Autodesk Fusion 360 part; units mm, degrees
(part 2 of 2)
sketch "スケッチ3" plane through (0, 0, 1.5) normal (0, 0, 1) x (-1, 0, 0)
  line L0 (-5.6421, -16.3724) -> (-10.7928, -25.2936)
  arc A0 (-10.7928, -25.2936) -> (-3.3, -27.3013) centre (0, 0) ccw
  line L1 (-3.3, -27.3013) -> (-3.3, -17)
  line L2 (-3.3, -17) -> (3.3, -17)
  line L3 (3.3, -17) -> (3.3, -27.3013)
  arc A1 (3.3, -27.3013) -> (10.7928, -25.2936) centre (0, 0) ccw
  line L4 (10.7928, -25.2936) -> (5.6421, -16.3724)
  line L5 (5.6421, -16.3724) -> (11.3579, -13.0724)
  line L6 (11.3579, -13.0724) -> (16.5085, -21.9936)
  arc A2 (16.5085, -21.9936) -> (21.9936, -16.5085) centre (0, 0) ccw
  line L7 (21.9936, -16.5085) -> (13.0724, -11.3579)
  line L8 (13.0724, -11.3579) -> (16.3724, -5.6421)
  line L9 (16.3724, -5.6421) -> (25.2936, -10.7928)
  arc A3 (25.2936, -10.7928) -> (27.3013, -3.3) centre (0, 0) ccw
  line L10 (27.3013, -3.3) -> (17, -3.3)
  line L11 (17, -3.3) -> (17, 3.3)
  line L12 (17, 3.3) -> (27.3013, 3.3)
  arc A4 (27.3013, 3.3) -> (25.2936, 10.7928) centre (0, 0) ccw
  line L13 (25.2936, 10.7928) -> (16.3724, 5.6421)
  line L14 (16.3724, 5.6421) -> (13.0724, 11.3579)
  line L15 (13.0724, 11.3579) -> (21.9936, 16.5085)
  arc A5 (21.9936, 16.5085) -> (16.5085, 21.9936) centre (0, 0) ccw
  line L16 (16.5085, 21.9936) -> (11.3579, 13.0724)
  line L17 (11.3579, 13.0724) -> (5.6421, 16.3724)
  line L18 (5.6421, 16.3724) -> (10.7928, 25.2936)
  arc A6 (10.7928, 25.2936) -> (3.3, 27.3013) centre (0, 0) ccw
  line L19 (3.3, 27.3013) -> (3.3, 17)
  line L20 (3.3, 17) -> (-3.3, 17)
  line L21 (-3.3, 17) -> (-3.3, 27.3013)
  arc A7 (-3.3, 27.3013) -> (-10.7928, 25.2936) centre (0, 0) ccw
  line L22 (-10.7928, 25.2936) -> (-5.6421, 16.3724)
  line L23 (-5.6421, 16.3724) -> (-11.3579, 13.0724)
  line L24 (-11.3579, 13.0724) -> (-16.5085, 21.9936)
  arc A8 (-16.5085, 21.9936) -> (-21.9936, 16.5085) centre (0, 0) ccw
  line L25 (-21.9936, 16.5085) -> (-13.0724, 11.3579)
  line L26 (-13.0724, 11.3579) -> (-16.3724, 5.6421)
  line L27 (-16.3724, 5.6421) -> (-25.2936, 10.7928)
  arc A9 (-25.2936, 10.7928) -> (-27.3013, 3.3) centre (0, 0) ccw
  line L28 (-27.3013, 3.3) -> (-17, 3.3)
  line L29 (-17, 3.3) -> (-17, -3.3)
  line L30 (-17, -3.3) -> (-27.3013, -3.3)
  arc A10 (-27.3013, -3.3) -> (-25.2936, -10.7928) centre (0, 0) ccw
  line L31 (-25.2936, -10.7928) -> (-16.3724, -5.6421)
  line L32 (-16.3724, -5.6421) -> (-13.0724, -11.3579)
  line L33 (-13.0724, -11.3579) -> (-21.9936, -16.5085)
  arc A11 (-21.9936, -16.5085) -> (-16.5085, -21.9936) centre (0, 0) ccw
  line L34 (-16.5085, -21.9936) -> (-11.3579, -13.0724)
  line L35 (-11.3579, -13.0724) -> (-5.6421, -16.3724)
  line L36 (3.3, -27.3013) -> (3.3, -26.1013)
  line L37 (3.3, -26.1013) -> (3.3, -23.5013)
  line L38 (3.3, -23.5013) -> (5.3, -23.5013)
  line L39 (5.3, -23.5013) -> (5.3, -26.1013)
  line L40 (5.3, -26.1013) -> (3.3, -26.1013)
  line L41 (3.3, -26.1013) -> (3.3, -23.5013)
  line L42 (-3.3, -27.3013) -> (-3.3, -26.1013)
  line L43 (-3.3, -26.1013) -> (-5.3, -26.1013)
  line L44 (-5.3, -26.1013) -> (-5.3, -23.5013)
  line L45 (-5.3, -23.5013) -> (-3.3, -23.5013)
  line L46 (-3.3, -23.5013) -> (-3.3, -26.1013)
  line L47 (14.6085, -18.7027) -> (16.3406, -17.7027)
  line L48 (16.3406, -17.7027) -> (17.6406, -19.9544)
  line L49 (17.6406, -19.9544) -> (15.9085, -20.9544)
  line L50 (15.9085, -20.9544) -> (14.6085, -18.7027)
  line L51 (8.8928, -22.0027) -> (10.1928, -24.2544)
  line L52 (7.1607, -23.0027) -> (8.8928, -22.0027)
  line L53 (8.4607, -25.2544) -> (7.1607, -23.0027)
  line L54 (10.1928, -24.2544) -> (8.4607, -25.2544)
  line L55 (22.0027, -8.8928) -> (23.0027, -7.1607)
  line L56 (23.0027, -7.1607) -> (25.2544, -8.4607)
  line L57 (25.2544, -8.4607) -> (24.2544, -10.1928)
  line L58 (24.2544, -10.1928) -> (22.0027, -8.8928)
  line L59 (18.7027, -14.6085) -> (20.9544, -15.9085)
  line L60 (17.7027, -16.3406) -> (18.7027, -14.6085)
  line L61 (19.9544, -17.6406) -> (17.7027, -16.3406)
  line L62 (20.9544, -15.9085) -> (19.9544, -17.6406)
  line L63 (23.5013, 3.3) -> (23.5013, 5.3)
  line L64 (23.5013, 5.3) -> (26.1013, 5.3)
  line L65 (26.1013, 5.3) -> (26.1013, 3.3)
  line L66 (26.1013, 3.3) -> (23.5013, 3.3)
  line L67 (23.5013, -3.3) -> (26.1013, -3.3)
  line L68 (23.5013, -5.3) -> (23.5013, -3.3)
  line L69 (26.1013, -5.3) -> (23.5013, -5.3)
  line L70 (26.1013, -3.3) -> (26.1013, -5.3)
  line L71 (18.7027, 14.6085) -> (17.7027, 16.3406)
  line L72 (17.7027, 16.3406) -> (19.9544, 17.6406)
  line L73 (19.9544, 17.6406) -> (20.9544, 15.9085)
  line L74 (20.9544, 15.9085) -> (18.7027, 14.6085)
  line L75 (22.0027, 8.8928) -> (24.2544, 10.1928)
  line L76 (23.0027, 7.1607) -> (22.0027, 8.8928)
  line L77 (25.2544, 8.4607) -> (23.0027, 7.1607)
  line L78 (24.2544, 10.1928) -> (25.2544, 8.4607)
  line L79 (8.8928, 22.0027) -> (7.1607, 23.0027)
  line L80 (7.1607, 23.0027) -> (8.4607, 25.2544)
  line L81 (8.4607, 25.2544) -> (10.1928, 24.2544)
  line L82 (10.1928, 24.2544) -> (8.8928, 22.0027)
  line L83 (14.6085, 18.7027) -> (15.9085, 20.9544)
  line L84 (16.3406, 17.7027) -> (14.6085, 18.7027)
  line L85 (17.6406, 19.9544) -> (16.3406, 17.7027)
  line L86 (15.9085, 20.9544) -> (17.6406, 19.9544)
  line L87 (-3.3, 23.5013) -> (-5.3, 23.5013)
  line L88 (-5.3, 23.5013) -> (-5.3, 26.1013)
  line L89 (-5.3, 26.1013) -> (-3.3, 26.1013)
  line L90 (-3.3, 26.1013) -> (-3.3, 23.5013)
  line L91 (3.3, 23.5013) -> (3.3, 26.1013)
  line L92 (5.3, 23.5013) -> (3.3, 23.5013)
  line L93 (5.3, 26.1013) -> (5.3, 23.5013)
  line L94 (3.3, 26.1013) -> (5.3, 26.1013)
  line L95 (-14.6085, 18.7027) -> (-16.3406, 17.7027)
  line L96 (-16.3406, 17.7027) -> (-17.6406, 19.9544)
  line L97 (-17.6406, 19.9544) -> (-15.9085, 20.9544)
  line L98 (-15.9085, 20.9544) -> (-14.6085, 18.7027)
  line L99 (-8.8928, 22.0027) -> (-10.1928, 24.2544)
  line L100 (-7.1607, 23.0027) -> (-8.8928, 22.0027)
  line L101 (-8.4607, 25.2544) -> (-7.1607, 23.0027)
  line L102 (-10.1928, 24.2544) -> (-8.4607, 25.2544)
  line L103 (-22.0027, 8.8928) -> (-23.0027, 7.1607)
  line L104 (-23.0027, 7.1607) -> (-25.2544, 8.4607)
  line L105 (-25.2544, 8.4607) -> (-24.2544, 10.1928)
  line L106 (-24.2544, 10.1928) -> (-22.0027, 8.8928)
  line L107 (-18.7027, 14.6085) -> (-20.9544, 15.9085)
  line L108 (-17.7027, 16.3406) -> (-18.7027, 14.6085)
  line L109 (-19.9544, 17.6406) -> (-17.7027, 16.3406)
  line L110 (-20.9544, 15.9085) -> (-19.9544, 17.6406)
  line L111 (-23.5013, -3.3) -> (-23.5013, -5.3)
  line L112 (-23.5013, -5.3) -> (-26.1013, -5.3)
  line L113 (-26.1013, -5.3) -> (-26.1013, -3.3)
  line L114 (-26.1013, -3.3) -> (-23.5013, -3.3)
  line L115 (-23.5013, 3.3) -> (-26.1013, 3.3)
  line L116 (-23.5013, 5.3) -> (-23.5013, 3.3)
  line L117 (-26.1013, 5.3) -> (-23.5013, 5.3)
  line L118 (-26.1013, 3.3) -> (-26.1013, 5.3)
  line L119 (-18.7027, -14.6085) -> (-17.7027, -16.3406)
  line L120 (-17.7027, -16.3406) -> (-19.9544, -17.6406)
  line L121 (-19.9544, -17.6406) -> (-20.9544, -15.9085)
  line L122 (-20.9544, -15.9085) -> (-18.7027, -14.6085)
  line L123 (-22.0027, -8.8928) -> (-24.2544, -10.1928)
  line L124 (-23.0027, -7.1607) -> (-22.0027, -8.8928)
  line L125 (-25.2544, -8.4607) -> (-23.0027, -7.1607)
  line L126 (-24.2544, -10.1928) -> (-25.2544, -8.4607)
  line L127 (-8.8928, -22.0027) -> (-7.1607, -23.0027)
  line L128 (-7.1607, -23.0027) -> (-8.4607, -25.2544)
  line L129 (-8.4607, -25.2544) -> (-10.1928, -24.2544)
  line L130 (-10.1928, -24.2544) -> (-8.8928, -22.0027)
  line L131 (-14.6085, -18.7027) -> (-15.9085, -20.9544)
  line L132 (-16.3406, -17.7027) -> (-14.6085, -18.7027)
  line L133 (-17.6406, -19.9544) -> (-16.3406, -17.7027)
  line L134 (-15.9085, -20.9544) -> (-17.6406, -19.9544)
  circle A12 centre (0, -6.25) radius 1.65
  circle A13 centre (5.4127, 3.125) radius 1.65
  circle A14 centre (-5.4127, 3.125) radius 1.65
  line L135 (4.752, 5.6303) -> (0, 2.8868)
  line L136 (0, 2.8868) -> (-4.752, 5.6303)
  line L137 (-4.752, 5.6303) -> (-6.2309, 14.1924)
  arc A15 (6.2309, 14.1924) -> (-6.2309, 14.1924) centre (0, 0) ccw
  line L138 (6.2309, 14.1924) -> (4.752, 5.6303)
  circle A16 centre (0, 0) radius 2.1
  arc A17 (15.4284, 1.4885) -> (9.0033, 12.6171) centre (0, 0) ccw
  line L139 (15.4284, 1.4885) -> (7.5798, 4.3762)
  line L140 (7.5798, 4.3762) -> (9.0033, 12.6171)
  line L141 (2.5, -6.9305) -> (2.5, -1.4434)
  line L142 (2.5, -1.4434) -> (7.252, 1.3002)
  line L143 (7.252, 1.3002) -> (15.4065, -1.7001)
  arc A18 (9.1755, -12.4924) -> (15.4065, -1.7001) centre (0, 0) ccw
  line L144 (9.1755, -12.4924) -> (2.5, -6.9305)
  arc A19 (-9.0033, 12.6171) -> (-15.4284, 1.4885) centre (0, 0) ccw
  line L145 (-9.0033, 12.6171) -> (-7.5798, 4.3762)
  line L146 (-7.5798, 4.3762) -> (-15.4284, 1.4885)
  line L147 (-6.4251, -14.1056) -> (0, -8.7524)
  line L148 (0, -8.7524) -> (6.4251, -14.1056)
  arc A20 (-6.4251, -14.1056) -> (6.4251, -14.1056) centre (0, 0) ccw
  line L149 (-2.5, -6.9305) -> (-9.1755, -12.4924)
  arc A21 (-15.4065, -1.7001) -> (-9.1755, -12.4924) centre (0, 0) ccw
  line L150 (-15.4065, -1.7001) -> (-7.252, 1.3002)
  line L151 (-7.252, 1.3002) -> (-2.5, -1.4434)
  line L152 (-2.5, -1.4434) -> (-2.5, -6.9305)
  dimension "d32" = 1.2
  dimension "d33" = 2.6
  dimension "d34" = 2
  dimension "d35" = 2.6
  dimension "d36" = 1.2
  dimension "d37" = 2
  dimension "d38" = 2.6
  dimension "d40" = 360
  constraint coincident L3.end A1.start
  constraint vertical L36
  constraint parallel L3 L37
  constraint horizontal L38
  constraint vertical L39
  constraint horizontal L40
  constraint vertical L41
  constraint coincident A0.end L1.start
  constraint parallel L1 L42
  constraint horizontal L43
  constraint vertical L44
  constraint horizontal L45
  constraint vertical L46
  measures "d32" distance of L3.end L36.end
  measures "d33" distance of L36.end L37.end
  measures "d34" distance of L37.end L38.end
  measures "d35" distance of L37.end L36.end
  measures "d36" distance of A0.end L42.end
  measures "d37" distance of L42.end L43.end
  measures "d38" distance of L42.end L45.end
extrude "押し出し3" add sketch "スケッチ3" along normal blind 0.5 contours L0 A0 L1 L2 L3 A1 L4 L5 L6 A2 L7 L8 L9 A3 L10 L11 L12 A4 L13 L14 L15 A5 L16 L17 L18 A6 L19 L20 L21 A7 L22 L23 L24 A8 L25 L26 L27 A9 L28 L29 L30 A10 L31 L32 L33 A11 L34 L35 L36 L38 L39 L40 L42 L43 L44 L45 L47 L48 L49 L52 L53 L54 L55 L56 L57 L60 L61 L62 L63 L64 L65 L68 L69 L70 L71 L72 L73 L76 L77 L78 L79 L80 L81 L84 L85 L86 L87 L88 L89 L92 L93 L94 L95 L96 L97 L100 L101 L102 L103 L104 L105 L108 L109 L110 L111 L112 L113 L116 L117 L118 L119 L120 L121 L124 L125 L126 L127 L128 L129 L132 L133 L134
extrude "押し出し4" cut 1 faces at (12.6956, -0.3629, 0) along direction (0, 0, 1) blind 0.5
fillet "フィレット1" radius 1.5 10 edges at (-9.1755, 12.4924, 1.25) (0, -2.8868, 1.25) (-2.5, 1.4434, 1.25) (-2.5, 6.9305, 1.25) (0, 8.7524, 1.25) (-6.4251, 14.1056, 1.25) (6.4251, 14.1056, 1.25) (9.1755, 12.4924, 1.25) (2.5, 6.9305, 1.25) (2.5, 1.4434, 1.25)
fillet "フィレット1" radius 1.5 14 edges at (-4.752, -5.6303, 1.25) (-7.5798, -4.3762, 1.25) (-7.252, -1.3002, 1.25) (-15.4284, -1.4885, 1.25) (-15.4065, 1.7001, 1.25) (-6.2309, -14.1924, 1.25) (-9.0033, -12.6171, 1.25) (6.2309, -14.1924, 1.25) (9.0033, -12.6171, 1.25) (4.752, -5.6303, 1.25) (15.4284, -1.4885, 1.25) (7.5798, -4.3762, 1.25) (7.252, -1.3002, 1.25) (15.4065, 1.7001, 1.25)
fillet "フィレット2" radius 0.5 4 edges at (17.7027, 16.3406, 1.75) (19.9544, 17.6406, 1.75) (23.0027, 7.1607, 1.75) (25.2544, 8.4607, 1.75)
fillet "フィレット3" radius 0.5 44 edges at (17.6406, 19.9544, 1.75) (16.3406, 17.7027, 1.75) (8.4607, 25.2544, 1.75) (5.3, 23.5013, 1.75) (7.1607, 23.0027, 1.75) (5.3, 26.1013, 1.75) (-5.3, 23.5013, 1.75) (-5.3, 26.1013, 1.75) (-8.4607, 25.2544, 1.75) (-7.1607, 23.0027, 1.75) (-17.6406, 19.9544, 1.75) (-16.3406, 17.7027, 1.75) (-19.9544, 17.6406, 1.75) (-17.7027, 16.3406, 1.75) (-25.2544, 8.4607, 1.75) (-23.0027, 7.1607, 1.75) (-23.5013, 5.3, 1.75) (-26.1013, 5.3, 1.75) (-26.1013, -5.3, 1.75) (-23.5013, -5.3, 1.75) (-23.0027, -7.1607, 1.75) (-25.2544, -8.4607, 1.75) (-17.7027, -16.3406, 1.75) (-16.3406, -17.7027, 1.75) (-19.9544, -17.6406, 1.75) (-17.6406, -19.9544, 1.75) (-7.1607, -23.0027, 1.75) (-5.3, -23.5013, 1.75) (-5.3, -26.1013, 1.75) (-8.4607, -25.2544, 1.75) (7.1607, -23.0027, 1.75) (5.3, -23.5013, 1.75) (8.4607, -25.2544, 1.75) (5.3, -26.1013, 1.75) (16.3406, -17.7027, 1.75) (17.7027, -16.3406, 1.75) (19.9544, -17.6406, 1.75) (17.6406, -19.9544, 1.75) (23.5013, -5.3, 1.75) (23.0027, -7.1607, 1.75) (25.2544, -8.4607, 1.75) (26.1013, -5.3, 1.75) (26.1013, 5.3, 1.75) (23.5013, 5.3, 1.75)
fillet "フィレット4" radius 1.5 24 edges at (13.0724, 11.3579, 1.25) (11.3579, 13.0724, 1.25) (5.6421, 16.3724, 1.25) (3.3, 17, 1.25) (-3.3, 17, 1.25) (-5.6421, 16.3724, 1.25) (-11.3579, 13.0724, 1.25) (-13.0724, 11.3579, 1.25) (-16.3724, 5.6421, 1.25) (-17, 3.3, 1.25) (-17, -3.3, 1.25) (-16.3724, -5.6421, 1.25) (-13.0724, -11.3579, 1.25) (-11.3579, -13.0724, 1.25) (-5.6421, -16.3724, 1.25) (-3.3, -17, 1.25) (3.3, -17, 1.25) (5.6421, -16.3724, 1.25) (13.0724, -11.3579, 1.25) (11.3579, -13.0724, 1.25) (17, -3.3, 1.25) (16.3724, -5.6421, 1.25) (17, 3.3, 1.25) (16.3724, 5.6421, 1.25)
extrude "押し出し5" add 1 faces at (6.483, -9.7763, 2) along direction (0, 0, 1) blind 2
extrude "押し出し6" cut 1 faces at (6.483, -9.7763, 4) along direction (0, 0, -1) blind 2

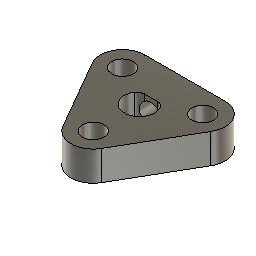
design "オムニ固定"
Autodesk Fusion 360 part; units mm, degrees
sketch "スケッチ1" plane through (0, 0, 0) normal (0, 0, 1) x (1, 0, 0)
  line L0 (2.5981, -7.75) -> (8.0107, 1.625)
  line L1 (0, -6.25) -> (5.4127, 3.125)
  circle A0 centre (5.4127, 3.125) radius 3
  line L2 (5.4127, 3.125) -> (8.0107, 1.625)
  line L3 (5.4127, 3.125) -> (5.4127, 6.125)
  line L4 (5.4127, 3.125) -> (-5.4127, 3.125)
  line L5 (-5.4127, 6.125) -> (5.4127, 6.125)
  circle A1 centre (-5.4127, 3.125) radius 3
  line L6 (-5.4127, 3.125) -> (0, -6.25)
  line L7 (-8.0107, 1.625) -> (-2.5981, -7.75)
  circle A2 centre (0, -6.25) radius 3
  line L8 (0, -6.25) -> (-2.5981, -7.75)
  line L9 (0, -6.25) -> (2.5981, -7.75)
  line L10 (-5.4127, 3.125) -> (-8.0107, 1.625)
  line L11 (-5.4127, 3.125) -> (-5.4127, 6.125)
  circle A3 centre (5.4127, 3.125) radius 1.45
  circle A4 centre (0, 0) radius 2.05
  circle A5 centre (0, -6.25) radius 1.45
  circle A6 centre (-5.4127, 3.125) radius 1.45
  line L12 (0, 0) -> (0, 1.53)
  line L13 (0, 1.53) -> (1.3644, 1.53)
  line L14 (0, 1.53) -> (-1.3644, 1.53)
  dimension "d1" = 6
  dimension "d2" = 6
  dimension "d3" = 6
  dimension "d4" = 2.9
  dimension "d5" = 4.1
  dimension "d6" = 2.9
  dimension "d9" = 2.9
  dimension "d13" = 1.53
  constraint coincident L1.start L6.end
  constraint coincident L1.end A0.centre
  constraint coincident L3.end A0
  constraint vertical L3
  constraint coincident L5.start A1
  constraint perpendicular L4 L11
  constraint coincident L0.end A0
  constraint perpendicular L1 L2
  constraint coincident L0.start A2
  constraint perpendicular L1 L9
  constraint coincident L7.end A2
  constraint perpendicular L6 L8
  constraint coincident L4.end A1.centre
  constraint coincident L7.start A1
  constraint parallel L8 L10
  constraint coincident A4.centre L12.start
  constraint concentric A2 A5
  constraint concentric A1 A6
  constraint vertical L12
  constraint coincident A4 L13.end
  constraint perpendicular L12 L13
  constraint coincident A4 L14.end
  constraint perpendicular L12 L14
  measures "d1" diameter of A2
  measures "d2" diameter of A0
  measures "d3" diameter of A1
  measures "d4" diameter of A3
  measures "d5" diameter of A4
  measures "d6" diameter of A5
  measures "d9" diameter of A6
  measures "d13" distance of A4.centre L12.end
extrude "押し出し1" add sketch "スケッチ1" along normal blind 4 contours L0 L1 A0 A2 | L1 A2 L9 A5 | A2 L8 L9 A5 | A0 L2 L3 A3 | L1 A0 L2 A3 | A1 L6 L7 A2 | L6 A2 L8 A5 | L1 A0 L4 A3 | L1 A0 L4 A1 L6 A2 | A1 L6 L10 A6 | A1 L10 L11 A6 | L1 L6 A2 A5 | A0 L3 L4 A3 | A0 L4 L5 A1 | L4 A1 L11 A6 | L4 A1 L6 A6 | A4 L13 L14 picked at (0.0992, 1.8694)
fillet "フィレット1" radius 0.97 2 edges at (-1.3644, 1.53, 2) (1.3644, 1.53, 2)
sketch "スケッチ2" plane through (0, 6.125, 0) normal (0, 1, 0) x (-1, 0, 0)
  line L0 (-5.4127, 0) -> (5.4127, 0)
  line L1 (5.4127, 0) -> (5.4127, 4)
  line L2 (5.4127, 4) -> (-5.4127, 4)
  line L3 (-5.4127, 4) -> (-5.4127, 0)
  line L4 (-5.4127, 4) -> (5.4127, 0)
  line L5 (-5.4127, 0) -> (5.4127, 4)
  circle A0 centre (0, 2) radius 1.45
  dimension "d16" = 2.9
  constraint coincident L2.end L3.start
  constraint coincident L0.end L1.start
  constraint coincident L0.start L3.end
  constraint coincident L1.end L2.start
  constraint midpoint L4 A0.centre
  measures "d16" diameter of A0
extrude "押し出し2" cut sketch "スケッチ2" against normal blind 7 contours L4 L5 A0 | L4 L5 A0 | L4 L5 A0 | L4 L5 A0

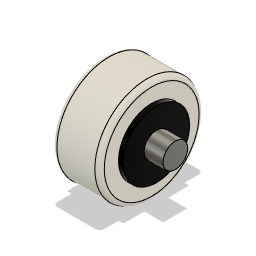
design "サイドホイール v1"
Autodesk Fusion 360 part; units mm, degrees
sketch "スケッチ1" plane through (0, 0, 0) normal (1, 0, 0) x (0, 0, -1)
  circle A0 centre (0, 0) radius 5.5
  circle A1 centre (0, 0) radius 2.5
  circle A2 centre (0, 0) radius 1.3
  circle A3 centre (0, 0) radius 3.5
  dimension "d1" = 11
  dimension "d2" = 5
  dimension "d7" = 2.6
  dimension "d14" = 7
  constraint coincident A0.centre A1.centre
  constraint concentric A0 A1
  constraint concentric A0 A2
  measures "d1" diameter of A0
  measures "d2" diameter of A1
  measures "d7" diameter of A2
  measures "d14" diameter of A3
extrude "押し出し1" add sketch "スケッチ1" along normal blind 5 contours A0 | A3 makes body 1
extrude "押し出し2" add sketch "スケッチ1" along normal blind 5 separate body contours A1 | A2 makes body 2
extrude "押し出し3" cut sketch "スケッチ1" along normal blind 16 contours A2 bodies 2
extrude "押し出し5" add sketch "スケッチ1" against normal blind 0.5 separate body contours A1 | A3 makes body 3
copy_body "ボディのコピーと貼り付け1" bodies 3 makes body 4
move_body "移動1" bodies 4 to x (1, 0, 0) y (0, 1, 0) z (0, 0, 1) at (5.5, 0, 0)
extrude "押し出し6" add sketch "スケッチ1" against normal blind 2.5 separate body contours A2 makes body 5
move_face "面をオフセット1" offset 7.5 1 faces at (0, 0.9052, 0.1692) on bodies 5
fillet "フィレット1" radius 0.5 1 edges at (0, -1.9889, 5.1278) on bodies 1
fillet "フィレット2" radius 0.5 1 edges at (5, -1.9889, 5.1278) on bodies 1

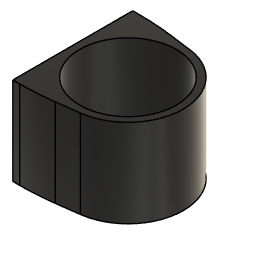
design "モーター固定具世界大会機"
Autodesk Fusion 360 part; units mm, degrees
sketch "スケッチ17" plane through (0, 0, 0) normal (0, 0, 1) x (1, 0, 0)
  circle A0 centre (0, 0) radius 11.6
  line L0 (0, 11.6) -> (0, 13.2)
  circle A1 centre (0, 0) radius 13.2
  circle A2 centre (0, 0) radius 7
  circle A3 centre (0, 0) radius 9
  circle A4 centre (0, 9) radius 1.1
  circle A5 centre (-6.364, 6.364) radius 1.1
  circle A6 centre (-9, 0) radius 1.1
  circle A7 centre (-6.364, -6.364) radius 1.1
  circle A8 centre (0, -9) radius 1.1
  circle A9 centre (6.364, -6.364) radius 1.1
  circle A10 centre (9, 0) radius 1.1
  circle A11 centre (6.364, 6.364) radius 1.1
  dimension "d120" = 23.2
  dimension "d121" = 1.6
  dimension "d122" = 14
  dimension "d123" = 18
  dimension "d124" = 2.2
  dimension "d126" = 360
  constraint coincident A0.centre A1.centre
  constraint coincident A0 L0.start
  constraint vertical L0
  constraint concentric A0 A1
  constraint coincident L0.end A1
  constraint coincident A3 A4.centre
  measures "d120" diameter of A0
  measures "d121" distance of L0.start L0.end
  measures "d122" diameter of A2
  measures "d123" diameter of A3
  measures "d124" diameter of A4
extrude "押し出し22" add sketch "スケッチ17" along normal blind 3 contours A0 | A1 | A3 A4 A5 A6 A7 A8 A9 A10 A11
sketch "スケッチ18" plane through (0, 0, 3) normal (0, 0, 1) x (-1, 0, 0)
  circle A0 centre (0, 9) radius 1.1
  circle A1 centre (6.364, -6.364) radius 1.1
  circle A2 centre (9, 0) radius 1.1
  circle A3 centre (0, -9) radius 1.1
  circle A4 centre (-6.364, -6.364) radius 1.1
  circle A5 centre (-9, 0) radius 1.1
  circle A6 centre (0, 0) radius 7
  circle A7 centre (-6.364, 6.364) radius 1.1
  circle A8 centre (6.364, 6.364) radius 1.1
  circle A9 centre (0, 0) radius 13.2
  circle A10 centre (0, 0) radius 11.7
  dimension "d129" = 23.4
  constraint concentric A6 A10
  measures "d129" diameter of A10
extrude "押し出し23" add sketch "スケッチ18" along normal blind 18 contours A9
sketch "スケッチ19" plane through (0, 0, 0) normal (1, 0, 0) x (0, 1, 0)
  line L0 (0, 0) -> (13.2, 0)
  line L1 (13.2, 0) -> (13.2, 21)
  line L2 (13.2, 21) -> (-13.2, 21)
  line L3 (-13.2, 21) -> (-13.2, 0)
  line L4 (-13.2, 0) -> (0, 0)
  line L5 (-13.2, 21) -> (-18.2, 21)
  line L6 (-18.2, 21) -> (-18.2, 0)
  line L7 (-18.2, 0) -> (-13.2, 0)
  line L8 (-13.2, 0) -> (-13.2, 21)
  line L9 (13.2, 21) -> (18.2, 21)
  line L10 (18.2, 21) -> (18.2, 0)
  line L11 (18.2, 0) -> (13.2, 0)
  line L12 (13.2, 0) -> (13.2, 21)
  dimension "d132" = 13.2
  dimension "d133" = 26.4
  dimension "d134" = 5
  dimension "d135" = 5
  constraint coincident L0.start L4.end
  constraint horizontal L0
  constraint perpendicular L0 L1
  constraint perpendicular L1 L2
  constraint perpendicular L0 L3
  constraint perpendicular L3 L4
  constraint horizontal L5
  constraint vertical L6
  constraint horizontal L7
  constraint vertical L8
  constraint horizontal L9
  constraint vertical L10
  constraint horizontal L11
  constraint vertical L12
  measures "d132" distance of L0.start L0.end
  measures "d133" distance of L1.end L2.end
  measures "d134" distance of L2.end L5.end
  measures "d135" distance of L1.end L9.end
extrude "押し出し24" add sketch "スケッチ19" against normal blind 13.2
sketch "スケッチ20" plane through (0, 0, 21) normal (0, 0, 1) x (-1, 0, 0)
  arc A0 (0, 13.2) -> (0, -13.2) centre (0, 0) ccw
  line L0 (0, -13.2) -> (0, -18.2)
  line L1 (0, -18.2) -> (13.2, -18.2)
  line L2 (13.2, -18.2) -> (13.2, 18.2)
  line L3 (13.2, 18.2) -> (0, 18.2)
  line L4 (0, 18.2) -> (0, 13.2)
  arc A1 (0, 11.7) -> (0, -11.7) centre (0, 0) ccw
  line L5 (0, 11.7) -> (0, -11.7)
  circle A2 centre (0, 0) radius 11.7
  constraint concentric A0 A2
  constraint coincident A1.start A2
extrude "押し出し25" cut sketch "スケッチ20" against normal blind 18 contours L5 A2
sketch "スケッチ22" plane through (0, 0, 21) normal (0, 0, 1) x (-1, 0, 0)
  circle A0 centre (0, 0) radius 11.7
  arc A1 (0, 13.2) -> (0, -13.2) centre (0, 0) ccw
  line L0 (0, -13.2) -> (0, -18.2)
  line L1 (0, -18.2) -> (13.2, -18.2)
  line L2 (13.2, -18.2) -> (13.2, 18.2)
  line L3 (13.2, 18.2) -> (0, 18.2)
  line L4 (0, 18.2) -> (0, 13.2)
  line L5 (13.2, 0) -> (7.2, 0)
  line L6 (7.2, 0) -> (7.2, 9.2223)
  line L7 (7.2, 9.2223) -> (13.2, 9.2223)
  line L8 (13.2, 9.2223) -> (13.2, 0)
  line L9 (7.2, 9.2223) -> (13.2, 9.2223)
  line L10 (13.2, 9.2223) -> (13.2, 14.2223)
  line L11 (13.2, 14.2223) -> (7.2, 14.2223)
  line L12 (7.2, 14.2223) -> (7.2, 9.2223)
  line L13 (13.2, 14.2223) -> (0, 14.2223)
  line L14 (-20, 0) -> (-2.5, 0)
  line L15 (7.2, -14.2223) -> (7.2, -9.2223)
  line L16 (7.2, -9.2223) -> (13.2, -9.2223)
  line L17 (13.2, -14.2223) -> (0, -14.2223)
  line L18 (13.2, -9.2223) -> (13.2, 0)
  line L19 (13.2, 0) -> (7.2, 0)
  line L20 (7.2, -9.2223) -> (13.2, -9.2223)
  line L21 (7.2, 0) -> (7.2, -9.2223)
  line L22 (13.2, -9.2223) -> (13.2, -14.2223)
  dimension "d140" = 6
  dimension "d141" = 5
  constraint horizontal L5
  constraint vertical L6
  constraint horizontal L7
  constraint vertical L8
  constraint coincident A0 L6.end
  constraint midpoint L2 L5.start
  constraint horizontal L9
  constraint vertical L10
  constraint horizontal L11
  constraint vertical L12
  constraint coincident L4 L13.end
  constraint perpendicular L4 L13
  constraint symmetric L5.start L14 L8.end
  constraint symmetric L5.end L14 L6.start
  constraint symmetric L6.end L14 L15.end
  constraint symmetric L7.end L14 L16.end
  constraint symmetric L10.end L14 L17.start
  constraint symmetric L11.end L14 L15.start
  constraint symmetric L13.end L14 L17.end
  measures "d140" distance of L5.start L5.end
  measures "d141" distance of L6.end L11.end
extrude "押し出し26" cut sketch "スケッチ22" against normal blind 21 contours L2 L3 L4 L11 L13 | L0 L1 L2 L17
sketch "スケッチ23" plane through (0, 0, 3) normal (0, 0, 1) x (-1, 0, 0)
  arc A0 (0, -7.9) -> (0, -10.1) centre (0, -9) ccw
  line L0 (0, -7.9) -> (0, -10.1)
  arc A1 (0, 7) -> (0, -7) centre (0, 0) ccw
  line L1 (0, 7) -> (0, -7)
  arc A2 (0, 10.1) -> (0, 7.9) centre (0, 9) ccw
  line L2 (0, 10.1) -> (0, 7.9)
  circle A3 centre (-6.364, 6.364) radius 1.1
  circle A4 centre (-9, 0) radius 1.1
  circle A5 centre (-6.364, -6.364) radius 1.1
  circle A6 centre (0, 0) radius 11.7
  circle A7 centre (0, 0) radius 7
  circle A8 centre (0, 9) radius 1.1
  circle A9 centre (-6.364, 6.364) radius 1.1
  circle A10 centre (-9, 0) radius 1.1
  circle A11 centre (-6.364, -6.364) radius 1.1
  circle A12 centre (0, -9) radius 1.1
  circle A13 centre (6.364, -6.364) radius 1.1
  circle A14 centre (9, 0) radius 1.1
  circle A15 centre (6.364, 6.364) radius 1.1
  dimension "d145" = 360
  constraint concentric A1 A7
  constraint coincident A1.start A7
  constraint concentric A2 A8
  constraint coincident A2.end A8
extrude "押し出し27" cut sketch "スケッチ23" against normal blind 3 contours L0 A12 | L1 A7 | L2 A8 | A13 | A14 | A15
sketch "スケッチ24" plane through (-13.2, 0, 0) normal (-1, 0, 0) x (0, -1, 0)
  line L0 (14.2223, 0) -> (14.2223, 21)
  line L1 (14.2223, 21) -> (-14.2223, 21)
  line L2 (-14.2223, 21) -> (-14.2223, 0)
  line L3 (-14.2223, 0) -> (14.2223, 0)
  line L4 (14.2223, 21) -> (11.2223, 21)
  line L5 (11.2223, 21) -> (11.2223, 16)
  line L6 (11.2223, 16) -> (14.2223, 16)
  line L7 (14.2223, 16) -> (14.2223, 21)
  line L8 (14.2223, 0) -> (11.2223, 0)
  line L9 (11.2223, 0) -> (11.2223, 3.4)
  line L10 (11.2223, 3.4) -> (14.2223, 3.4)
  line L11 (14.2223, 3.4) -> (14.2223, 0)
  line L12 (-14.2223, 0) -> (-11.2223, 0)
  line L13 (-11.2223, 0) -> (-11.2223, 3.4)
  line L14 (-11.2223, 3.4) -> (-14.2223, 3.4)
  line L15 (-14.2223, 3.4) -> (-14.2223, 0)
  line L16 (-14.2223, 21) -> (-11.2223, 21)
  line L17 (-11.2223, 21) -> (-11.2223, 16)
  line L18 (-11.2223, 16) -> (-14.2223, 16)
  line L19 (-14.2223, 16) -> (-14.2223, 21)
  circle A0 centre (11.2223, 3.4) radius 2.35
  circle A1 centre (11.2223, 16) radius 2.35
  circle A2 centre (-11.2223, 3.4) radius 2.35
  circle A3 centre (-11.2223, 16) radius 2.35
  dimension "d148" = 3
  dimension "d149" = 5
  dimension "d150" = 3
  dimension "d151" = 3.4
  dimension "d152" = 3
  dimension "d153" = 3.4
  dimension "d154" = 3
  dimension "d155" = 5
  dimension "d156" = 4.7
  dimension "d157" = 4.7
  dimension "d158" = 4.7
  dimension "d159" = 4.7
  constraint horizontal L4
  constraint vertical L5
  constraint horizontal L6
  constraint vertical L7
  constraint coincident L0.end L1.start
  constraint horizontal L8
  constraint vertical L9
  constraint horizontal L10
  constraint vertical L11
  constraint coincident L0.start L3.end
  constraint horizontal L12
  constraint vertical L13
  constraint horizontal L14
  constraint vertical L15
  constraint coincident L2.end L3.start
  constraint horizontal L16
  constraint vertical L17
  constraint horizontal L18
  constraint vertical L19
  constraint coincident L1.end L2.start
  constraint coincident L9.end L10.start
  constraint coincident L5.end L6.start
  constraint coincident L13.end L14.start
  constraint coincident L17.end L18.start
  measures "d148" distance of L0.end L4.end
  measures "d149" distance of L0.end L6.end
  measures "d150" distance of L0.start L8.end
  measures "d151" distance of L0.start L10.end
  measures "d152" distance of L2.end L12.end
  measures "d153" distance of L2.end L14.end
  measures "d154" distance of L1.end L16.end
  measures "d155" distance of L1.end L18.end
  measures "d156" diameter of A0
  measures "d157" diameter of A1
  measures "d158" diameter of A2
  measures "d159" diameter of A3
extrude "押し出し28" cut sketch "スケッチ24" against normal blind 5.5 contours L9 L10 A0 | L9 L10 A0 | L5 L6 A1 | L5 L6 A1 | L13 L14 A2 | L13 L14 A2 | L17 L18 A3 | L17 L18 A3
extrude "押し出し29" add 1 faces at (-8.8, -14.2223, 7) along direction (0, -1, 0) blind 0.1
extrude "押し出し30" add 1 faces at (-8.8, 14.2223, 7) along direction (0, 1, 0) blind 0.1
fillet "フィレット2" radius 60 2 edges at (0, 14.3223, 10.5) (0, -14.3223, 10.5)
fillet "フィレット3" radius 2025 2 edges at (0, 13.2, 10.5) (0, -13.2, 10.5)
sketch "スケッチ26" plane through (0, 0, 21) normal (0, 0, 1) x (-1, 0, 0)
  arc A0 (-1.7185, 13.0877) -> (-1.7185, -13.0877) centre (0, 0) ccw
  arc A1 (3.5819, -13.7908) -> (-1.7185, -13.0877) centre (-265.3548, -2020.8528) ccw
  arc A2 (3.5819, -13.7908) -> (11.5504, -14.3223) centre (11.5504, 45.6777) ccw
  line L0 (11.5504, -14.3223) -> (13.2, -14.3223)
  line L1 (13.2, -14.3223) -> (13.2, 14.3223)
  line L2 (13.2, 14.3223) -> (11.5504, 14.3223)
  arc A3 (11.5504, 14.3223) -> (3.5819, 13.7908) centre (11.5504, -45.6777) ccw
  arc A4 (-1.7185, 13.0877) -> (3.5819, 13.7908) centre (-265.3548, 2020.8528) ccw
  circle A5 centre (0, 0) radius 11.7
  circle A6 centre (0, 0) radius 11.55
  circle A7 centre (0, 0) radius 11.7
  dimension "d176" = 23.1
  constraint coincident A0.centre A5.centre
  constraint concentric A6 A7
  measures "d176" diameter of A6
extrude "押し出し31" add sketch "スケッチ26" against normal blind 21 contours A5 A7
